Autodesk Fusion 360 part; units mm, degrees
(part 5 of 8)
  spline S134 degree 5 poles (58.96, -141.4145) (58.9068, -141.4906) (58.8007, -141.6428) (58.6419, -141.8712) (58.4312, -142.1762) (58.1694, -142.5582) (57.9092, -142.9408) (57.6506, -143.324) (57.3936, -143.708) (57.1382, -144.0925) (56.8845, -144.4778) (56.6323, -144.8637) (56.3819, -145.2503) (56.1331, -145.6375) (55.8859, -146.0254) (55.6405, -146.4139) (55.3968, -146.8031) (55.1548, -147.193) (54.9146, -147.5836) (54.6761, -147.9747) (54.4394, -148.3666) (54.2045, -148.7591) (53.9713, -149.1523) (53.74, -149.5462) (53.5106, -149.9407) (53.2829, -150.3358) (53.0572, -150.7317) (52.8333, -151.1282) (52.6114, -151.5253) (52.3914, -151.9232) (52.1734, -152.3217) (51.9573, -152.7208) (51.7432, -153.1207) (51.5311, -153.5212) (51.3211, -153.9223) (51.1132, -154.3242) (50.9074, -154.7267) (50.7037, -155.1299) (50.5021, -155.5337) (50.3027, -155.9383) (50.1056, -156.3435) (49.9107, -156.7494) (49.718, -157.156) (49.5277, -157.5633) (49.3397, -157.9713) (49.1542, -158.3799) (48.9711, -158.7893) (48.7905, -159.1994) (48.6124, -159.6102) (48.4369, -160.0216) (48.2641, -160.4338) (48.0939, -160.8467) (47.9263, -161.2604) (47.7616, -161.6747) (47.5997, -162.0898) (47.4409, -162.5056) (47.2851, -162.9223) (47.1327, -163.3396) (46.9836, -163.7578) (46.8379, -164.1768) (46.6955, -164.5965) (46.5565, -165.0171) (46.4209, -165.4384) (46.3021, -165.8187) (46.2122, -166.1152) (46.1493, -166.3273) (46.1121, -166.4549) (46.0997, -166.4977) knots -1 -1 -1 -1 -1 -1 -0.98571429 -0.97142857 -0.95714286 -0.94285714 -0.92857143 -0.91428571 -0.9 -0.88571429 -0.87142857 -0.85714286 -0.84285714 -0.82857143 -0.81428571 -0.8 -0.78571429 -0.77142857 -0.75714286 -0.74285714 -0.72857143 -0.71428571 -0.7 -0.68571429 -0.67142857 -0.65714286 -0.64285714 -0.62857143 -0.61428571 -0.6 -0.58571429 -0.57142857 -0.55714286 -0.54285714 -0.52857143 -0.51428571 -0.5 -0.48571429 -0.47142857 -0.45714286 -0.44285714 -0.42857143 -0.41428571 -0.4 -0.38571429 -0.37142857 -0.35714286 -0.34285714 -0.32857143 -0.31428571 -0.3 -0.28571429 -0.27142857 -0.25714286 -0.24285714 -0.22857143 -0.21428571 -0.2 -0.18571429 -0.17142857 -0.15714286 -0.14285714 -0.12857143 -0.11428571 -0.10707295 -0.10707295 -0.10707295 -0.10707295 -0.10707295 -0.10707295
  spline S135 degree 3 poles (44.3847, -167.6316) (44.5899, -167.6564) (44.798, -167.6408) (45.1965, -167.5309) (45.3832, -167.4375) (45.6787, -167.2088) (45.7938, -167.0864) (45.9817, -166.8102) (46.0532, -166.6581) (46.0997, -166.4977) knots 0 0 0 0 0.062015 0.062015 0.12403 0.12403 0.174133 0.174133 0.224236 0.224236 0.224236 0.224236
  arc A68 (44.3847, -167.6316) -> (36.0479, -166.7554) centre (11.949, -436.1388) ccw
  spline S136 degree 3 poles (34.6061, -165.2897) (34.6211, -165.4958) (34.6763, -165.6971) (34.8607, -166.0671) (34.9881, -166.2324) (35.2693, -166.4786) (35.4115, -166.5681) (35.7186, -166.6994) (35.8816, -166.7405) (36.0479, -166.7554) knots 0 0 0 0 0.062015 0.062015 0.12403 0.12403 0.174133 0.174133 0.224236 0.224236 0.224236 0.224236
  spline S137 degree 5 poles (34.6061, -165.2897) (34.6029, -165.2452) (34.593, -165.1127) (34.5756, -164.8921) (34.5493, -164.5834) (34.5122, -164.1867) (34.4672, -163.7464) (34.4186, -163.3062) (34.3666, -162.866) (34.3112, -162.4259) (34.2523, -161.9859) (34.19, -161.5459) (34.1243, -161.106) (34.0553, -160.6662) (33.9833, -160.2266) (33.9083, -159.787) (33.8304, -159.3476) (33.7498, -158.9083) (33.6664, -158.4692) (33.5803, -158.0302) (33.4916, -157.5914) (33.4002, -157.1527) (33.3062, -156.7143) (33.2096, -156.2759) (33.1106, -155.8378) (33.0091, -155.3998) (32.9052, -154.9621) (32.7989, -154.5245) (32.6903, -154.0872) (32.5794, -153.65) (32.4663, -153.2131) (32.3508, -152.7763) (32.2332, -152.3398) (32.1134, -151.9035) (31.9913, -151.4674) (31.8672, -151.0316) (31.7409, -150.596) (31.6125, -150.1606) (31.4821, -149.7255) (31.3496, -149.2906) (31.2151, -148.856) (31.0786, -148.4216) (30.9401, -147.9875) (30.7996, -147.5536) (30.6572, -147.12) (30.5128, -146.6867) (30.3665, -146.2537) (30.2183, -145.8209) (30.0683, -145.3884) (29.9163, -144.9561) (29.7625, -144.5242) (29.6069, -144.0925) (29.4494, -143.6611) (29.2902, -143.23) (29.1291, -142.7993) (28.9662, -142.3688) (28.8016, -141.9386) (28.6352, -141.5087) (28.4671, -141.0791) (28.2973, -140.6498) (28.1257, -140.2208) (27.9524, -139.7922) (27.7774, -139.3639) (27.6008, -138.9358) (27.4581, -138.5937) (27.3503, -138.3372) (27.2781, -138.1663) (27.242, -138.0808) knots 0.10707295 0.10707295 0.10707295 0.10707295 0.10707295 0.10707295 0.11428571 0.12857143 0.14285714 0.15714286 0.17142857 0.18571429 0.2 0.21428571 0.22857143 0.24285714 0.25714286 0.27142857 0.28571429 0.3 0.31428571 0.32857143 0.34285714 0.35714286 0.37142857 0.38571429 0.4 0.41428571 0.42857143 0.44285714 0.45714286 0.47142857 0.48571429 0.5 0.51428571 0.52857143 0.54285714 0.55714286 0.57142857 0.58571429 0.6 0.61428571 0.62857143 0.64285714 0.65714286 0.67142857 0.68571429 0.7 0.71428571 0.72857143 0.74285714 0.75714286 0.77142857 0.78571429 0.8 0.81428571 0.82857143 0.84285714 0.85714286 0.87142857 0.88571429 0.9 0.91428571 0.92857143 0.94285714 0.95714286 0.97142857 0.98571429 1 1 1 1 1 1
  arc A69 (27.242, -138.0808) -> (17.4848, -137.7401) centre (11.949, -436.1388) ccw
  spline S138 degree 5 poles (17.4848, -137.7401) (17.4427, -137.8228) (17.3588, -137.9883) (17.2334, -138.2366) (17.0672, -138.568) (16.8611, -138.9826) (16.6567, -139.3977) (16.4539, -139.8132) (16.2528, -140.2292) (16.0535, -140.6456) (15.8558, -141.0624) (15.6598, -141.4796) (15.4656, -141.8973) (15.2731, -142.3154) (15.0824, -142.7339) (14.8934, -143.1528) (14.7063, -143.5722) (14.5209, -143.9919) (14.3373, -144.4121) (14.1556, -144.8327) (13.9757, -145.2537) (13.7977, -145.6751) (13.6216, -146.0969) (13.4473, -146.5191) (13.275, -146.9417) (13.1046, -147.3647) (12.9361, -147.7881) (12.7697, -148.2119) (12.6052, -148.6361) (12.4427, -149.0606) (12.2822, -149.4856) (12.1238, -149.9109) (11.9674, -150.3367) (11.8132, -150.7628) (11.661, -151.1893) (11.511, -151.6162) (11.3632, -152.0434) (11.2176, -152.471) (11.0742, -152.899) (10.9331, -153.3274) (10.7943, -153.7561) (10.6578, -154.1852) (10.5236, -154.6146) (10.3918, -155.0444) (10.2624, -155.4746) (10.1355, -155.9051) (10.0112, -156.336) (9.8894, -156.7672) (9.7702, -157.1988) (9.6537, -157.6307) (9.5399, -158.0629) (9.4289, -158.4955) (9.3205, -158.9284) (9.2151, -159.3616) (9.1125, -159.7952) (9.0131, -160.2291) (8.9169, -160.6633) (8.824, -161.0979) (8.7345, -161.5327) (8.6485, -161.9679) (8.566, -162.4034) (8.4868, -162.8392) (8.4112, -163.2752) (8.3465, -163.6684) (8.2987, -163.9745) (8.266, -164.1933) (8.2469, -164.3248) (8.2406, -164.369) knots -1 -1 -1 -1 -1 -1 -0.98571429 -0.97142857 -0.95714286 -0.94285714 -0.92857143 -0.91428571 -0.9 -0.88571429 -0.87142857 -0.85714286 -0.84285714 -0.82857143 -0.81428571 -0.8 -0.78571429 -0.77142857 -0.75714286 -0.74285714 -0.72857143 -0.71428571 -0.7 -0.68571429 -0.67142857 -0.65714286 -0.64285714 -0.62857143 -0.61428571 -0.6 -0.58571429 -0.57142857 -0.55714286 -0.54285714 -0.52857143 -0.51428571 -0.5 -0.48571429 -0.47142857 -0.45714286 -0.44285714 -0.42857143 -0.41428571 -0.4 -0.38571429 -0.37142857 -0.35714286 -0.34285714 -0.32857143 -0.31428571 -0.3 -0.28571429 -0.27142857 -0.25714286 -0.24285714 -0.22857143 -0.21428571 -0.2 -0.18571429 -0.17142857 -0.15714286 -0.14285714 -0.12857143 -0.11428571 -0.10707295 -0.10707295 -0.10707295 -0.10707295 -0.10707295 -0.10707295
  spline S139 degree 3 poles (6.7, -165.7305) (6.9067, -165.7265) (7.1106, -165.6821) (7.49, -165.5178) (7.6618, -165.3994) (7.9226, -165.1317) (8.0196, -164.9945) (8.1672, -164.6948) (8.2168, -164.5343) (8.2406, -164.369) knots 0 0 0 0 0.062015 0.062015 0.12403 0.12403 0.174133 0.174133 0.224236 0.224236 0.224236 0.224236
  arc A70 (6.7, -165.7305) -> (-1.6775, -166.0231) centre (11.949, -436.1388) ccw
  spline S140 degree 3 poles (-3.3093, -164.7723) (-3.2657, -164.9744) (-3.1831, -165.166) (-2.949, -165.5068) (-2.7998, -165.6527) (-2.4871, -165.8573) (-2.3338, -165.9262) (-2.0114, -166.0135) (-1.8443, -166.0315) (-1.6775, -166.0231) knots 0 0 0 0 0.062015 0.062015 0.12403 0.12403 0.174133 0.174133 0.224236 0.224236 0.224236 0.224236
  spline S141 degree 5 poles (-3.3093, -164.7723) (-3.3187, -164.7287) (-3.3469, -164.5989) (-3.3948, -164.3828) (-3.4638, -164.0808) (-3.5558, -163.6931) (-3.6617, -163.2634) (-3.771, -162.8342) (-3.8838, -162.4055) (-3.9999, -161.9774) (-4.1195, -161.5499) (-4.2424, -161.1229) (-4.3687, -160.6964) (-4.4982, -160.2705) (-4.6307, -159.8451) (-4.7661, -159.4203) (-4.9044, -158.996) (-5.0454, -158.5722) (-5.1891, -158.149) (-5.3354, -157.7263) (-5.4844, -157.3041) (-5.6359, -156.8824) (-5.7901, -156.4612) (-5.9467, -156.0406) (-6.1057, -155.6205) (-6.2672, -155.201) (-6.431, -154.7819) (-6.5971, -154.3634) (-6.7655, -153.9454) (-6.9362, -153.528) (-7.109, -153.111) (-7.2841, -152.6946) (-7.4614, -152.2787) (-7.6408, -151.8633) (-7.8223, -151.4485) (-8.0059, -151.0342) (-8.1916, -150.6204) (-8.3793, -150.2071) (-8.569, -149.7944) (-8.7607, -149.3822) (-8.9544, -148.9705) (-9.15, -148.5593) (-9.3476, -148.1487) (-9.5471, -147.7386) (-9.7485, -147.3291) (-9.9518, -146.9201) (-10.1569, -146.5116) (-10.3639, -146.1036) (-10.5727, -145.6962) (-10.7833, -145.2893) (-10.9957, -144.883) (-11.2099, -144.4772) (-11.4259, -144.0719) (-11.6436, -143.6672) (-11.8631, -143.263) (-12.0843, -142.8594) (-12.3071, -142.4563) (-12.5317, -142.0537) (-12.758, -141.6517) (-12.986, -141.2502) (-13.2156, -140.8493) (-13.4468, -140.449) (-13.6797, -140.0492) (-13.9142, -139.6499) (-14.1031, -139.3309) (-14.2455, -139.0919) (-14.3408, -138.9327) (-14.3885, -138.8531) knots 0.10707295 0.10707295 0.10707295 0.10707295 0.10707295 0.10707295 0.11428571 0.12857143 0.14285714 0.15714286 0.17142857 0.18571429 0.2 0.21428571 0.22857143 0.24285714 0.25714286 0.27142857 0.28571429 0.3 0.31428571 0.32857143 0.34285714 0.35714286 0.37142857 0.38571429 0.4 0.41428571 0.42857143 0.44285714 0.45714286 0.47142857 0.48571429 0.5 0.51428571 0.52857143 0.54285714 0.55714286 0.57142857 0.58571429 0.6 0.61428571 0.62857143 0.64285714 0.65714286 0.67142857 0.68571429 0.7 0.71428571 0.72857143 0.74285714 0.75714286 0.77142857 0.78571429 0.8 0.81428571 0.82857143 0.84285714 0.85714286 0.87142857 0.88571429 0.9 0.91428571 0.92857143 0.94285714 0.95714286 0.97142857 0.98571429 1 1 1 1 1 1
  arc A71 (-14.3885, -138.8531) -> (-24.0982, -139.8737) centre (11.949, -436.1388) ccw
  spline S142 degree 5 poles (-24.0982, -139.8737) (-24.1283, -139.9614) (-24.1884, -140.137) (-24.278, -140.4003) (-24.3965, -140.7516) (-24.5428, -141.1909) (-24.6875, -141.6304) (-24.8305, -142.0701) (-24.9717, -142.51) (-25.1112, -142.9501) (-25.2489, -143.3903) (-25.3849, -143.8308) (-25.5191, -144.2714) (-25.6516, -144.7122) (-25.7822, -145.1532) (-25.911, -145.5944) (-26.038, -146.0357) (-26.1631, -146.4771) (-26.2864, -146.9188) (-26.4078, -147.3605) (-26.5274, -147.8025) (-26.645, -148.2445) (-26.7607, -148.6868) (-26.8745, -149.1291) (-26.9864, -149.5716) (-27.0962, -150.0142) (-27.2041, -150.4569) (-27.31, -150.8997) (-27.4139, -151.3427) (-27.5157, -151.7858) (-27.6155, -152.2289) (-27.7131, -152.6722) (-27.8087, -153.1155) (-27.9022, -153.559) (-27.9935, -154.0025) (-28.0826, -154.4461) (-28.1695, -154.8897) (-28.2542, -155.3335) (-28.3366, -155.7772) (-28.4167, -156.2211) (-28.4945, -156.6649) (-28.57, -157.1088) (-28.6431, -157.5528) (-28.7138, -157.9968) (-28.7821, -158.4407) (-28.8478, -158.8847) (-28.911, -159.3287) (-28.9716, -159.7727) (-29.0295, -160.2166) (-29.0847, -160.6605) (-29.1373, -161.1044) (-29.1871, -161.5482) (-29.2341, -161.992) (-29.2783, -162.4357) (-29.3195, -162.8793) (-29.3576, -163.3228) (-29.3924, -163.7662) (-29.4239, -164.2095) (-29.452, -164.6525) (-29.4766, -165.0954) (-29.4977, -165.5382) (-29.5154, -165.9807) (-29.5296, -166.4231) (-29.539, -166.8215) (-29.5437, -167.1312) (-29.5456, -167.3525) (-29.5462, -167.4853) (-29.5464, -167.5299) knots -1 -1 -1 -1 -1 -1 -0.98571429 -0.97142857 -0.95714286 -0.94285714 -0.92857143 -0.91428571 -0.9 -0.88571429 -0.87142857 -0.85714286 -0.84285714 -0.82857143 -0.81428571 -0.8 -0.78571429 -0.77142857 -0.75714286 -0.74285714 -0.72857143 -0.71428571 -0.7 -0.68571429 -0.67142857 -0.65714286 -0.64285714 -0.62857143 -0.61428571 -0.6 -0.58571429 -0.57142857 -0.55714286 -0.54285714 -0.52857143 -0.51428571 -0.5 -0.48571429 -0.47142857 -0.45714286 -0.44285714 -0.42857143 -0.41428571 -0.4 -0.38571429 -0.37142857 -0.35714286 -0.34285714 -0.32857143 -0.31428571 -0.3 -0.28571429 -0.27142857 -0.25714286 -0.24285714 -0.22857143 -0.21428571 -0.2 -0.18571429 -0.17142857 -0.15714286 -0.14285714 -0.12857143 -0.11428571 -0.10707295 -0.10707295 -0.10707295 -0.10707295 -0.10707295 -0.10707295
  spline S143 degree 3 poles (-30.8825, -169.0926) (-30.6783, -169.0599) (-30.4826, -168.9876) (-30.1298, -168.772) (-29.9761, -168.6308) (-29.7551, -168.3295) (-29.6782, -168.1801) (-29.5737, -167.8628) (-29.5469, -167.6969) (-29.5464, -167.5299) knots 0 0 0 0 0.062015 0.062015 0.12403 0.12403 0.174133 0.174133 0.224236 0.224236 0.224236 0.224236
  arc A72 (-30.8825, -169.0926) -> (-39.1377, -170.5482) centre (11.949, -436.1388) ccw
  spline S144 degree 3 poles (-40.9277, -169.5368) (-40.8564, -169.7308) (-40.7479, -169.9091) (-40.4687, -170.2139) (-40.3007, -170.3377) (-39.9625, -170.4968) (-39.8011, -170.5436) (-39.4697, -170.5853) (-39.3017, -170.5798) (-39.1377, -170.5482) knots 0 0 0 0 0.062015 0.062015 0.12403 0.12403 0.174133 0.174133 0.224236 0.224236 0.224236 0.224236
  spline S145 degree 5 poles (-40.9277, -169.5368) (-40.9431, -169.4949) (-40.9891, -169.3703) (-41.0666, -169.163) (-41.177, -168.8735) (-41.322, -168.5024) (-41.4866, -168.0916) (-41.6547, -167.6818) (-41.826, -167.273) (-42.0006, -166.8652) (-42.1785, -166.4585) (-42.3597, -166.0527) (-42.5441, -165.648) (-42.7315, -165.2442) (-42.922, -164.8415) (-43.1152, -164.4396) (-43.3112, -164.0387) (-43.5098, -163.6386) (-43.711, -163.2395) (-43.9147, -162.8413) (-44.121, -162.4439) (-44.3298, -162.0474) (-44.541, -161.6519) (-44.7546, -161.2571) (-44.9706, -160.8633) (-45.1889, -160.4703) (-45.4094, -160.0781) (-45.6322, -159.6868) (-45.8571, -159.2963) (-46.0842, -158.9066) (-46.3134, -158.5178) (-46.5448, -158.1298) (-46.7782, -157.7426) (-47.0136, -157.3562) (-47.2511, -156.9707) (-47.4906, -156.586) (-47.732, -156.202) (-47.9754, -155.8189) (-48.2208, -155.4366) (-48.468, -155.0551) (-48.7171, -154.6744) (-48.968, -154.2945) (-49.2208, -153.9153) (-49.4755, -153.537) (-49.7319, -153.1595) (-49.9901, -152.7827) (-50.2501, -152.4068) (-50.5119, -152.0316) (-50.7753, -151.6572) (-51.0405, -151.2836) (-51.3074, -150.9108) (-51.576, -150.5387) (-51.8463, -150.1674) (-52.1182, -149.797) (-52.3918, -149.4273) (-52.667, -149.0583) (-52.9438, -148.6902) (-53.2222, -148.3228) (-53.5022, -147.9562) (-53.7838, -147.5904) (-54.067, -147.2253) (-54.3517, -146.861) (-54.638, -146.4975) (-54.9258, -146.1348) (-55.1572, -145.8452) (-55.3315, -145.6283) (-55.448, -145.4839) (-55.5064, -145.4118) knots 0.10707295 0.10707295 0.10707295 0.10707295 0.10707295 0.10707295 0.11428571 0.12857143 0.14285714 0.15714286 0.17142857 0.18571429 0.2 0.21428571 0.22857143 0.24285714 0.25714286 0.27142857 0.28571429 0.3 0.31428571 0.32857143 0.34285714 0.35714286 0.37142857 0.38571429 0.4 0.41428571 0.42857143 0.44285714 0.45714286 0.47142857 0.48571429 0.5 0.51428571 0.52857143 0.54285714 0.55714286 0.57142857 0.58571429 0.6 0.61428571 0.62857143 0.64285714 0.65714286 0.67142857 0.68571429 0.7 0.71428571 0.72857143 0.74285714 0.75714286 0.77142857 0.78571429 0.8 0.81428571 0.82857143 0.84285714 0.85714286 0.87142857 0.88571429 0.9 0.91428571 0.92857143 0.94285714 0.95714286 0.97142857 0.98571429 1 1 1 1 1 1
  arc A73 (-55.5064, -145.4118) -> (-64.9795, -147.7737) centre (11.949, -436.1388) ccw
  spline S146 degree 5 poles (-64.9795, -147.7737) (-64.9971, -147.8648) (-65.0322, -148.047) (-65.0843, -148.3203) (-65.1527, -148.6846) (-65.2365, -149.14) (-65.3186, -149.5954) (-65.399, -150.0507) (-65.4776, -150.5059) (-65.5545, -150.9611) (-65.6296, -151.4163) (-65.703, -151.8714) (-65.7746, -152.3264) (-65.8444, -152.7814) (-65.9123, -153.2362) (-65.9785, -153.691) (-66.0428, -154.1457) (-66.1053, -154.6003) (-66.1659, -155.0548) (-66.2247, -155.5092) (-66.2816, -155.9634) (-66.3365, -156.4176) (-66.3896, -156.8716) (-66.4407, -157.3254) (-66.4899, -157.7792) (-66.5371, -158.2328) (-66.5823, -158.6862) (-66.6255, -159.1395) (-66.6668, -159.5926) (-66.7059, -160.0455) (-66.743, -160.4982) (-66.7781, -160.9508) (-66.811, -161.4031) (-66.8418, -161.8552) (-66.8705, -162.3071) (-66.897, -162.7588) (-66.9214, -163.2102) (-66.9435, -163.6614) (-66.9633, -164.1124) (-66.9809, -164.563) (-66.9962, -165.0134) (-67.0092, -165.4635) (-67.0198, -165.9133) (-67.028, -166.3628) (-67.0338, -166.8119) (-67.0371, -167.2608) (-67.0379, -167.7092) (-67.0361, -168.1573) (-67.0316, -168.605) (-67.0246, -169.0522) (-67.0148, -169.4991) (-67.0024, -169.9456) (-66.9872, -170.3916) (-66.9692, -170.8371) (-66.9482, -171.2821) (-66.9242, -171.7266) (-66.897, -172.1706) (-66.8665, -172.6139) (-66.8326, -173.0565) (-66.7953, -173.4985) (-66.7547, -173.9399) (-66.7106, -174.3806) (-66.6631, -174.8207) (-66.617, -175.2164) (-66.5785, -175.5238) (-66.5496, -175.7432) (-66.5317, -175.8749) (-66.5257, -175.919) knots -1 -1 -1 -1 -1 -1 -0.98571429 -0.97142857 -0.95714286 -0.94285714 -0.92857143 -0.91428571 -0.9 -0.88571429 -0.87142857 -0.85714286 -0.84285714 -0.82857143 -0.81428571 -0.8 -0.78571429 -0.77142857 -0.75714286 -0.74285714 -0.72857143 -0.71428571 -0.7 -0.68571429 -0.67142857 -0.65714286 -0.64285714 -0.62857143 -0.61428571 -0.6 -0.58571429 -0.57142857 -0.55714286 -0.54285714 -0.52857143 -0.51428571 -0.5 -0.48571429 -0.47142857 -0.45714286 -0.44285714 -0.42857143 -0.41428571 -0.4 -0.38571429 -0.37142857 -0.35714286 -0.34285714 -0.32857143 -0.31428571 -0.3 -0.28571429 -0.27142857 -0.25714286 -0.24285714 -0.22857143 -0.21428571 -0.2 -0.18571429 -0.17142857 -0.15714286 -0.14285714 -0.12857143 -0.11428571 -0.10707295 -0.10707295 -0.10707295 -0.10707295 -0.10707295 -0.10707295
  spline S147 degree 3 poles (-67.6313, -177.6525) (-67.4337, -177.5917) (-67.2499, -177.4928) (-66.9305, -177.2303) (-66.798, -177.0691) (-66.6211, -176.7399) (-66.5657, -176.5812) (-66.5064, -176.2525) (-66.5029, -176.0845) (-66.5257, -175.919) knots 0 0 0 0 0.062015 0.062015 0.12403 0.12403 0.174133 0.174133 0.224236 0.224236 0.224236 0.224236
  arc A74 (-67.6313, -177.6525) -> (-75.6036, -180.2429) centre (11.949, -436.1388) ccw
  spline S148 degree 3 poles (-77.517, -179.4903) (-77.4194, -179.6726) (-77.2871, -179.834) (-76.9682, -180.097) (-76.7845, -180.1962) (-76.4275, -180.3067) (-76.2612, -180.3306) (-75.9272, -180.3257) (-75.7616, -180.2969) (-75.6036, -180.2429) knots 0 0 0 0 0.062015 0.062015 0.12403 0.12403 0.174133 0.174133 0.224236 0.224236 0.224236 0.224236
  spline S149 degree 5 poles (-77.517, -179.4903) (-77.538, -179.451) (-77.6009, -179.334) (-77.7065, -179.1395) (-77.8561, -178.8683) (-78.0514, -178.5209) (-78.2716, -178.137) (-78.495, -177.7546) (-78.7215, -177.3736) (-78.9512, -176.9941) (-79.184, -176.6161) (-79.4198, -176.2395) (-79.6588, -175.8644) (-79.9006, -175.4906) (-80.1453, -175.1183) (-80.3926, -174.7472) (-80.6424, -174.3775) (-80.8948, -174.009) (-81.1495, -173.6417) (-81.4067, -173.2757) (-81.6663, -172.9109) (-81.9282, -172.5474) (-82.1924, -172.185) (-82.4589, -171.8239) (-82.7276, -171.4639) (-82.9985, -171.1051) (-83.2714, -170.7474) (-83.5465, -170.3909) (-83.8236, -170.0355) (-84.1027, -169.6813) (-84.3838, -169.3281) (-84.6669, -168.9761) (-84.9519, -168.6252) (-85.2388, -168.2754) (-85.5277, -167.9266) (-85.8184, -167.579) (-86.1109, -167.2324) (-86.4052, -166.8869) (-86.7014, -166.5424) (-86.9993, -166.199) (-87.2989, -165.8567) (-87.6003, -165.5154) (-87.9034, -165.1751) (-88.2083, -164.8359) (-88.5147, -164.4977) (-88.8229, -164.1606) (-89.1327, -163.8245) (-89.4441, -163.4894) (-89.7571, -163.1553) (-90.0717, -162.8222) (-90.3879, -162.4902) (-90.7056, -162.1591) (-91.0249, -161.8291) (-91.3458, -161.5001) (-91.6681, -161.172) (-91.992, -160.845) (-92.3174, -160.5189) (-92.6442, -160.1939) (-92.9725, -159.8698) (-93.3023, -159.5467) (-93.6335, -159.2246) (-93.9662, -158.9035) (-94.3002, -158.5834) (-94.6357, -158.2642) (-94.9052, -158.0097) (-95.108, -157.8192) (-95.2435, -157.6924) (-95.3113, -157.6291) knots 0.10707295 0.10707295 0.10707295 0.10707295 0.10707295 0.10707295 0.11428571 0.12857143 0.14285714 0.15714286 0.17142857 0.18571429 0.2 0.21428571 0.22857143 0.24285714 0.25714286 0.27142857 0.28571429 0.3 0.31428571 0.32857143 0.34285714 0.35714286 0.37142857 0.38571429 0.4 0.41428571 0.42857143 0.44285714 0.45714286 0.47142857 0.48571429 0.5 0.51428571 0.52857143 0.54285714 0.55714286 0.57142857 0.58571429 0.6 0.61428571 0.62857143 0.64285714 0.65714286 0.67142857 0.68571429 0.7 0.71428571 0.72857143 0.74285714 0.75714286 0.77142857 0.78571429 0.8 0.81428571 0.82857143 0.84285714 0.85714286 0.87142857 0.88571429 0.9 0.91428571 0.92857143 0.94285714 0.95714286 0.97142857 0.98571429 1 1 1 1 1 1
  arc A75 (-95.3113, -157.6291) -> (-104.3635, -161.2864) centre (11.949, -436.1388) ccw
  spline S150 degree 5 poles (-104.3635, -161.2864) (-104.3683, -161.3791) (-104.3776, -161.5644) (-104.3912, -161.8423) (-104.4082, -162.2126) (-104.4278, -162.6752) (-104.4458, -163.1376) (-104.462, -163.5996) (-104.4765, -164.0614) (-104.4893, -164.5229) (-104.5003, -164.9841) (-104.5097, -165.4449) (-104.5172, -165.9055) (-104.523, -166.3657) (-104.527, -166.8256) (-104.5293, -167.2852) (-104.5297, -167.7444) (-104.5283, -168.2033) (-104.5251, -168.6618) (-104.52, -169.1199) (-104.5131, -169.5777) (-104.5043, -170.035) (-104.4937, -170.492) (-104.4811, -170.9486) (-104.4667, -171.4047) (-104.4503, -171.8605) (-104.432, -172.3158) (-104.4117, -172.7707) (-104.3895, -173.2251) (-104.3652, -173.6791) (-104.339, -174.1325) (-104.3107, -174.5856) (-104.2803, -175.0381) (-104.248, -175.4901) (-104.2135, -175.9416) (-104.1769, -176.3926) (-104.1381, -176.843) (-104.0972, -177.2929) (-104.0541, -177.7422) (-104.0088, -178.1909) (-103.9613, -178.639) (-103.9115, -179.0865) (-103.8594, -179.5334) (-103.8049, -179.9797) (-103.7482, -180.4253) (-103.689, -180.8702) (-103.6273, -181.3144) (-103.5632, -181.7579) (-103.4965, -182.2006) (-103.4273, -182.6425) (-103.3554, -183.0837) (-103.281, -183.524) (-103.2038, -183.9636) (-103.124, -184.4023) (-103.0413, -184.8401) (-102.9557, -185.2769) (-102.8669, -185.7127) (-102.7751, -186.1475) (-102.6799, -186.5811) (-102.5815, -187.0136) (-102.4798, -187.4451) (-102.3748, -187.8753) (-102.2665, -188.3045) (-102.1657, -188.69) (-102.0849, -188.989) (-102.0258, -189.2023) (-101.9897, -189.3302) (-101.9775, -189.373) knots -1 -1 -1 -1 -1 -1 -0.98571429 -0.97142857 -0.95714286 -0.94285714 -0.92857143 -0.91428571 -0.9 -0.88571429 -0.87142857 -0.85714286 -0.84285714 -0.82857143 -0.81428571 -0.8 -0.78571429 -0.77142857 -0.75714286 -0.74285714 -0.72857143 -0.71428571 -0.7 -0.68571429 -0.67142857 -0.65714286 -0.64285714 -0.62857143 -0.61428571 -0.6 -0.58571429 -0.57142857 -0.55714286 -0.54285714 -0.52857143 -0.51428571 -0.5 -0.48571429 -0.47142857 -0.45714286 -0.44285714 -0.42857143 -0.41428571 -0.4 -0.38571429 -0.37142857 -0.35714286 -0.34285714 -0.32857143 -0.31428571 -0.3 -0.28571429 -0.27142857 -0.25714286 -0.24285714 -0.22857143 -0.21428571 -0.2 -0.18571429 -0.17142857 -0.15714286 -0.14285714 -0.12857143 -0.11428571 -0.10707295 -0.10707295 -0.10707295 -0.10707295 -0.10707295 -0.10707295
  spline S151 degree 3 poles (-102.8311, -191.2435) (-102.644, -191.1558) (-102.4757, -191.0323) (-102.196, -190.7279) (-102.0872, -190.5498) (-101.9578, -190.1992) (-101.925, -190.0344) (-101.9121, -189.7006) (-101.932, -189.5337) (-101.9775, -189.373) knots 0 0 0 0 0.062015 0.062015 0.12403 0.12403 0.174133 0.174133 0.224236 0.224236 0.224236 0.224236
  arc A76 (-102.8311, -191.2435) -> (-110.3654, -194.9182) centre (11.949, -436.1388) ccw
  spline S152 degree 3 poles (-112.3648, -194.4393) (-112.2428, -194.6061) (-112.0894, -194.7476) (-111.737, -194.9637) (-111.5413, -195.0363) (-111.1724, -195.0961) (-111.0043, -195.0966) (-110.6743, -195.0453) (-110.5144, -194.9937) (-110.3654, -194.9182) knots 0 0 0 0 0.062015 0.062015 0.12403 0.12403 0.174133 0.174133 0.224236 0.224236 0.224236 0.224236
  spline S153 degree 5 poles (-112.3648, -194.4393) (-112.3912, -194.4033) (-112.4697, -194.2961) (-112.6013, -194.1183) (-112.7872, -193.8704) (-113.029, -193.5537) (-113.3005, -193.2041) (-113.5749, -192.8565) (-113.8523, -192.5108) (-114.1325, -192.1669) (-114.4156, -191.825) (-114.7016, -191.4849) (-114.9905, -191.1467) (-115.282, -190.8102) (-115.576, -190.4756) (-115.8726, -190.1425) (-116.1715, -189.8111) (-116.4726, -189.4814) (-116.776, -189.1531) (-117.0817, -188.8265) (-117.3895, -188.5014) (-117.6994, -188.1778) (-118.0115, -187.8558) (-118.3257, -187.5352) (-118.6418, -187.2161) (-118.96, -186.8985) (-119.2801, -186.5823) (-119.6021, -186.2676) (-119.9259, -185.9542) (-120.2516, -185.6422) (-120.5791, -185.3317) (-120.9085, -185.0225) (-121.2396, -184.7146) (-121.5724, -184.4081) (-121.907, -184.103) (-122.2432, -183.7991) (-122.5811, -183.4966) (-122.9207, -183.1955) (-123.2619, -182.8956) (-123.6047, -182.597) (-123.9491, -182.2997) (-124.295, -182.0036) (-124.6425, -181.7089) (-124.9916, -181.4154) (-125.3422, -181.1232) (-125.6942, -180.8322) (-126.0478, -180.5425) (-126.4028, -180.254) (-126.7592, -179.9667) (-127.1171, -179.6807) (-127.4765, -179.3958) (-127.8372, -179.1122) (-128.1993, -178.8299) (-128.5628, -178.5487) (-128.9277, -178.2687) (-129.2939, -177.9899) (-129.6615, -177.7123) (-130.0304, -177.4359) (-130.4007, -177.1607) (-130.7722, -176.8867) (-131.145, -176.6138) (-131.5191, -176.3421) (-131.8945, -176.0716) (-132.2711, -175.8022) (-132.5734, -175.5877) (-132.8007, -175.4273) (-132.9525, -175.3206) (-133.0285, -175.2673) knots 0.10707295 0.10707295 0.10707295 0.10707295 0.10707295 0.10707295 0.11428571 0.12857143 0.14285714 0.15714286 0.17142857 0.18571429 0.2 0.21428571 0.22857143 0.24285714 0.25714286 0.27142857 0.28571429 0.3 0.31428571 0.32857143 0.34285714 0.35714286 0.37142857 0.38571429 0.4 0.41428571 0.42857143 0.44285714 0.45714286 0.47142857 0.48571429 0.5 0.51428571 0.52857143 0.54285714 0.55714286 0.57142857 0.58571429 0.6 0.61428571 0.62857143 0.64285714 0.65714286 0.67142857 0.68571429 0.7 0.71428571 0.72857143 0.74285714 0.75714286 0.77142857 0.78571429 0.8 0.81428571 0.82857143 0.84285714 0.85714286 0.87142857 0.88571429 0.9 0.91428571 0.92857143 0.94285714 0.95714286 0.97142857 0.98571429 1 1 1 1 1 1
  arc A77 (-133.0285, -175.2673) -> (-141.4836, -180.1488) centre (11.949, -436.1388) ccw
  spline S154 degree 5 poles (-141.4836, -180.1488) (-141.4754, -180.2413) (-141.4589, -180.4261) (-141.4337, -180.7031) (-141.399, -181.0722) (-141.354, -181.5331) (-141.3075, -181.9934) (-141.2592, -182.4532) (-141.2093, -182.9125) (-141.1577, -183.3713) (-141.1045, -183.8295) (-141.0496, -184.2872) (-140.993, -184.7444) (-140.9347, -185.2009) (-140.8746, -185.6569) (-140.8129, -186.1123) (-140.7494, -186.5671) (-140.6841, -187.0213) (-140.6172, -187.4749) (-140.5484, -187.9279) (-140.4778, -188.3802) (-140.4055, -188.8319) (-140.3314, -189.283) (-140.2554, -189.7333) (-140.1776, -190.1831) (-140.0979, -190.6321) (-140.0164, -191.0804) (-139.9331, -191.528) (-139.8478, -191.9749) (-139.7606, -192.4211) (-139.6715, -192.8665) (-139.5804, -193.3112) (-139.4874, -193.7551) (-139.3924, -194.1982) (-139.2954, -194.6405) (-139.1964, -195.082) (-139.0954, -195.5227) (-138.9922, -195.9625) (-138.887, -196.4014) (-138.7797, -196.8394) (-138.6703, -197.2766) (-138.5587, -197.7128) (-138.4449, -198.1481) (-138.3289, -198.5825) (-138.2106, -199.0158) (-138.0901, -199.4481) (-137.9672, -199.8794) (-137.842, -200.3097) (-137.7144, -200.7388) (-137.5843, -201.1668) (-137.4518, -201.5937) (-137.3167, -202.0194) (-137.1792, -202.4439) (-137.039, -202.8672) (-136.8962, -203.2892) (-136.7506, -203.7099) (-136.6021, -204.1291) (-136.4506, -204.5469) (-136.296, -204.9631) (-136.1384, -205.3777) (-135.9776, -205.7907) (-135.8138, -206.2022) (-135.6468, -206.6121) (-135.4934, -206.9799) (-135.3717, -207.2647) (-135.2835, -207.4677) (-135.23, -207.5893) (-135.212, -207.6301) knots -1 -1 -1 -1 -1 -1 -0.98571429 -0.97142857 -0.95714286 -0.94285714 -0.92857143 -0.91428571 -0.9 -0.88571429 -0.87142857 -0.85714286 -0.84285714 -0.82857143 -0.81428571 -0.8 -0.78571429 -0.77142857 -0.75714286 -0.74285714 -0.72857143 -0.71428571 -0.7 -0.68571429 -0.67142857 -0.65714286 -0.64285714 -0.62857143 -0.61428571 -0.6 -0.58571429 -0.57142857 -0.55714286 -0.54285714 -0.52857143 -0.51428571 -0.5 -0.48571429 -0.47142857 -0.45714286 -0.44285714 -0.42857143 -0.41428571 -0.4 -0.38571429 -0.37142857 -0.35714286 -0.34285714 -0.32857143 -0.31428571 -0.3 -0.28571429 -0.27142857 -0.25714286 -0.24285714 -0.22857143 -0.21428571 -0.2 -0.18571429 -0.17142857 -0.15714286 -0.14285714 -0.12857143 -0.11428571 -0.10707295 -0.10707295 -0.10707295 -0.10707295 -0.10707295 -0.10707295
  spline S155 degree 3 poles (-135.7969, -209.6011) (-135.6238, -209.4882) (-135.4744, -209.3425) (-135.2397, -209.0021) (-135.1568, -208.8106) (-135.0774, -208.4454) (-135.0679, -208.2776) (-135.1016, -207.9453) (-135.1445, -207.7828) (-135.212, -207.6301) knots 0 0 0 0 0.062015 0.062015 0.12403 0.12403 0.174133 0.174133 0.224236 0.224236 0.224236 0.224236
  arc A78 (-135.7969, -209.6011) -> (-142.7465, -214.2886) centre (11.949, -436.1388) ccw
  spline S156 degree 3 poles (-144.7931, -214.0926) (-144.6491, -214.2409) (-144.4774, -214.3596) (-144.0983, -214.5246) (-143.8945, -214.5692) (-143.5208, -214.5771) (-143.3544, -214.5542) (-143.0347, -214.4574) (-142.8835, -214.3841) (-142.7465, -214.2886) knots 0 0 0 0 0.062015 0.062015 0.12403 0.12403 0.174133 0.174133 0.224236 0.224236 0.224236 0.224236
  spline S157 degree 5 poles (-144.7931, -214.0926) (-144.8242, -214.0606) (-144.9169, -213.9655) (-145.072, -213.8076) (-145.2905, -213.5881) (-145.574, -213.3081) (-145.8915, -212.9997) (-146.2117, -212.6937) (-146.5344, -212.3899) (-146.8598, -212.0884) (-147.1878, -211.7892) (-147.5183, -211.4922) (-147.8514, -211.1975) (-148.1869, -210.9049) (-148.5247, -210.6144) (-148.8647, -210.3259) (-149.2068, -210.0393) (-149.5509, -209.7546) (-149.897, -209.4719) (-150.2452, -209.1909) (-150.5952, -208.9118) (-150.9472, -208.6345) (-151.3011, -208.3591) (-151.6568, -208.0853) (-152.0143, -207.8134) (-152.3735, -207.5431) (-152.7345, -207.2746) (-153.0972, -207.0077) (-153.4615, -206.7424) (-153.8274, -206.4788) (-154.195, -206.2168) (-154.5641, -205.9565) (-154.9349, -205.6977) (-155.3071, -205.4405) (-155.6809, -205.1849) (-156.0561, -204.9308) (-156.4329, -204.6783) (-156.811, -204.4273) (-157.1907, -204.1778) (-157.5717, -203.9299) (-157.9541, -203.6834) (-158.3379, -203.4384) (-158.723, -203.1949) (-159.1095, -202.9528) (-159.4974, -202.7122) (-159.8865, -202.4731) (-160.2769, -202.2353) (-160.6686, -201.9991) (-161.0616, -201.7642) (-161.4558, -201.5308) (-161.8513, -201.2987) (-162.248, -201.0681) (-162.6459, -200.8388) (-163.045, -200.611) (-163.4453, -200.3845) (-163.8468, -200.1594) (-164.2494, -199.9357) (-164.6532, -199.7133) (-165.0581, -199.4923) (-165.4641, -199.2726) (-165.8713, -199.0543) (-166.2796, -198.8373) (-166.6889, -198.6217) (-167.0994, -198.4074) (-167.4286, -198.237) (-167.6761, -198.1098) (-167.8412, -198.0252) (-167.9238, -197.983) knots 0.10707295 0.10707295 0.10707295 0.10707295 0.10707295 0.10707295 0.11428571 0.12857143 0.14285714 0.15714286 0.17142857 0.18571429 0.2 0.21428571 0.22857143 0.24285714 0.25714286 0.27142857 0.28571429 0.3 0.31428571 0.32857143 0.34285714 0.35714286 0.37142857 0.38571429 0.4 0.41428571 0.42857143 0.44285714 0.45714286 0.47142857 0.48571429 0.5 0.51428571 0.52857143 0.54285714 0.55714286 0.57142857 0.58571429 0.6 0.61428571 0.62857143 0.64285714 0.65714286 0.67142857 0.68571429 0.7 0.71428571 0.72857143 0.74285714 0.75714286 0.77142857 0.78571429 0.8 0.81428571 0.82857143 0.84285714 0.85714286 0.87142857 0.88571429 0.9 0.91428571 0.92857143 0.94285714 0.95714286 0.97142857 0.98571429 1 1 1 1 1 1
  arc A79 (-167.9238, -197.983) -> (-175.6173, -203.9938) centre (11.949, -436.1388) ccw
  spline S158 degree 5 poles (-175.6173, -203.9938) (-175.5964, -204.0842) (-175.5543, -204.2649) (-175.4907, -204.5357) (-175.405, -204.8964) (-175.2964, -205.3465) (-175.1862, -205.7959) (-175.0744, -206.2445) (-174.9611, -206.6924) (-174.8462, -207.1396) (-174.7297, -207.5859) (-174.6116, -208.0315) (-174.4919, -208.4763) (-174.3706, -208.9203) (-174.2477, -209.3635) (-174.1232, -209.8059) (-173.997, -210.2474) (-173.8692, -210.6881) (-173.7397, -211.128) (-173.6086, -211.567) (-173.4758, -212.0051) (-173.3413, -212.4423) (-173.2051, -212.8787) (-173.0672, -213.3141) (-172.9275, -213.7486) (-172.7862, -214.1822) (-172.6431, -214.6148) (-172.4982, -215.0465) (-172.3515, -215.4772) (-172.2031, -215.9068) (-172.0529, -216.3355) (-171.9008, -216.7632) (-171.7469, -217.1898) (-171.5912, -217.6154) (-171.4336, -218.0399) (-171.2741, -218.4633) (-171.1127, -218.8856) (-170.9494, -219.3068) (-170.7841, -219.7268) (-170.6169, -220.1457) (-170.4476, -220.5633) (-170.2764, -220.9798) (-170.1031, -221.395) (-169.9278, -221.809) (-169.7504, -222.2217) (-169.5709, -222.633) (-169.3892, -223.043) (-169.2053, -223.4516) (-169.0192, -223.8588) (-168.8308, -224.2645) (-168.6402, -224.6688) (-168.4472, -225.0716) (-168.2519, -225.4728) (-168.0542, -225.8725) (-167.8541, -226.2706) (-167.6513, -226.6669) (-167.4459, -227.0614) (-167.2378, -227.4539) (-167.0268, -227.8446) (-166.8129, -228.2332) (-166.5963, -228.6199) (-166.3768, -229.0046) (-166.1544, -229.3872) (-165.9512, -229.73) (-165.7911, -229.9952) (-165.6755, -230.1839) (-165.6056, -230.2969) (-165.5821, -230.3347) knots -1 -1 -1 -1 -1 -1 -0.98571429 -0.97142857 -0.95714286 -0.94285714 -0.92857143 -0.91428571 -0.9 -0.88571429 -0.87142857 -0.85714286 -0.84285714 -0.82857143 -0.81428571 -0.8 -0.78571429 -0.77142857 -0.75714286 -0.74285714 -0.72857143 -0.71428571 -0.7 -0.68571429 -0.67142857 -0.65714286 -0.64285714 -0.62857143 -0.61428571 -0.6 -0.58571429 -0.57142857 -0.55714286 -0.54285714 -0.52857143 -0.51428571 -0.5 -0.48571429 -0.47142857 -0.45714286 -0.44285714 -0.42857143 -0.41428571 -0.4 -0.38571429 -0.37142857 -0.35714286 -0.34285714 -0.32857143 -0.31428571 -0.3 -0.28571429 -0.27142857 -0.25714286 -0.24285714 -0.22857143 -0.21428571 -0.2 -0.18571429 -0.17142857 -0.15714286 -0.14285714 -0.12857143 -0.11428571 -0.10707295 -0.10707295 -0.10707295 -0.10707295 -0.10707295 -0.10707295
  spline S159 degree 3 poles (-165.887, -232.368) (-165.7313, -232.2321) (-165.6036, -232.067) (-165.4186, -231.6973) (-165.3631, -231.4961) (-165.3353, -231.1234) (-165.3493, -230.956) (-165.4289, -230.6316) (-165.494, -230.4766) (-165.5821, -230.3347) knots 0 0 0 0 0.062015 0.062015 0.12403 0.12403 0.174133 0.174133 0.224236 0.224236 0.224236 0.224236
  arc A80 (-165.887, -232.368) -> (-172.1165, -237.9771) centre (11.949, -436.1388) ccw
  spline S160 degree 3 poles (-174.1705, -238.0678) (-174.0073, -238.1946) (-173.8208, -238.2883) (-173.4224, -238.3989) (-173.2143, -238.4148) (-172.8432, -238.3705) (-172.6816, -238.3247) (-172.3785, -238.1844) (-172.2389, -238.0907) (-172.1165, -237.9771) knots 0 0 0 0 0.062015 0.062015 0.12403 0.12403 0.174133 0.174133 0.224236 0.224236 0.224236 0.224236
  spline S161 degree 5 poles (-174.1705, -238.0678) (-174.2058, -238.0405) (-174.3108, -237.9592) (-174.4864, -237.8245) (-174.7334, -237.6375) (-175.053, -237.3996) (-175.4104, -237.1384) (-175.77, -236.8799) (-176.1319, -236.624) (-176.4961, -236.3708) (-176.8625, -236.1201) (-177.2312, -235.872) (-177.602, -235.6265) (-177.975, -235.3835) (-178.3499, -235.1428) (-178.7267, -234.9044) (-179.1054, -234.6682) (-179.4858, -234.4342) (-179.8679, -234.2024) (-180.2517, -233.9726) (-180.6372, -233.745) (-181.0244, -233.5194) (-181.4131, -233.2958) (-181.8035, -233.0743) (-182.1954, -232.8547) (-182.5887, -232.6371) (-182.9836, -232.4214) (-183.3798, -232.2075) (-183.7775, -231.9956) (-184.1766, -231.7855) (-184.577, -231.5772) (-184.9788, -231.3708) (-185.382, -231.1661) (-185.7864, -230.9632) (-186.1921, -230.7621) (-186.599, -230.5627) (-187.0073, -230.3651) (-187.4167, -230.1692) (-187.8273, -229.975) (-188.2391, -229.7824) (-188.6521, -229.5916) (-189.0663, -229.4024) (-189.4816, -229.2148) (-189.898, -229.0289) (-190.3155, -228.8446) (-190.7342, -228.662) (-191.1539, -228.4809) (-191.5747, -228.3014) (-191.9965, -228.1235) (-192.4194, -227.9472) (-192.8433, -227.7725) (-193.2682, -227.5993) (-193.6942, -227.4277) (-194.1211, -227.2576) (-194.549, -227.089) (-194.9779, -226.922) (-195.4078, -226.7565) (-195.8386, -226.5925) (-196.2703, -226.43) (-196.703, -226.2689) (-197.1366, -226.1094) (-197.571, -225.9514) (-198.0064, -225.7948) (-198.4427, -225.6397) (-198.7925, -225.5167) (-199.0552, -225.4252) (-199.2305, -225.3645) (-199.3182, -225.3342) knots 0.10707295 0.10707295 0.10707295 0.10707295 0.10707295 0.10707295 0.11428571 0.12857143 0.14285714 0.15714286 0.17142857 0.18571429 0.2 0.21428571 0.22857143 0.24285714 0.25714286 0.27142857 0.28571429 0.3 0.31428571 0.32857143 0.34285714 0.35714286 0.37142857 0.38571429 0.4 0.41428571 0.42857143 0.44285714 0.45714286 0.47142857 0.48571429 0.5 0.51428571 0.52857143 0.54285714 0.55714286 0.57142857 0.58571429 0.6 0.61428571 0.62857143 0.64285714 0.65714286 0.67142857 0.68571429 0.7 0.71428571 0.72857143 0.74285714 0.75714286 0.77142857 0.78571429 0.8 0.81428571 0.82857143 0.84285714 0.85714286 0.87142857 0.88571429 0.9 0.91428571 0.92857143 0.94285714 0.95714286 0.97142857 0.98571429 1 1 1 1 1 1
  arc A81 (-199.3182, -225.3342) -> (-206.1003, -232.3572) centre (11.949, -436.1388) ccw
  spline S162 degree 5 poles (-206.1003, -232.3572) (-206.0669, -232.4438) (-206.0001, -232.6169) (-205.8995, -232.8763) (-205.7644, -233.2215) (-205.5942, -233.6521) (-205.4225, -234.0818) (-205.2494, -234.5105) (-205.0748, -234.9382) (-204.8988, -235.365) (-204.7213, -235.7908) (-204.5424, -236.2157) (-204.362, -236.6395) (-204.1801, -237.0623) (-203.9967, -237.484) (-203.8118, -237.9048) (-203.6254, -238.3245) (-203.4375, -238.7431) (-203.248, -239.1606) (-203.0571, -239.5771) (-202.8646, -239.9925) (-202.6706, -240.4067) (-202.475, -240.8199) (-202.2778, -241.2319) (-202.079, -241.6427) (-201.8787, -242.0524) (-201.6768, -242.4609) (-201.4733, -242.8682) (-201.2681, -243.2743) (-201.0613, -243.6791) (-200.8529, -244.0828) (-200.6428, -244.4851) (-200.431, -244.8862) (-200.2176, -245.2859) (-200.0024, -245.6844) (-199.7855, -246.0815) (-199.5669, -246.4772) (-199.3466, -246.8715) (-199.1245, -247.2645) (-198.9006, -247.656) (-198.6749, -248.046) (-198.4473, -248.4346) (-198.218, -248.8216) (-197.9868, -249.2072) (-197.7537, -249.5912) (-197.5186, -249.9735) (-197.2816, -250.3542) (-197.0427, -250.7333) (-196.8017, -251.1106) (-196.5587, -251.4862) (-196.3136, -251.86) (-196.0665, -252.232) (-195.8172, -252.6022) (-195.5659, -252.9704) (-195.3122, -253.3368) (-195.0563, -253.701) (-194.798, -254.063) (-194.5373, -254.4228) (-194.2739, -254.7803) (-194.0081, -255.1354) (-193.7397, -255.4881) (-193.4688, -255.8385) (-193.1953, -256.1865) (-192.9465, -256.4977) (-192.751, -256.738) (-192.6102, -256.9088) (-192.5253, -257.0109) (-192.4967, -257.0452) knots -1 -1 -1 -1 -1 -1 -0.98571429 -0.97142857 -0.95714286 -0.94285714 -0.92857143 -0.91428571 -0.9 -0.88571429 -0.87142857 -0.85714286 -0.84285714 -0.82857143 -0.81428571 -0.8 -0.78571429 -0.77142857 -0.75714286 -0.74285714 -0.72857143 -0.71428571 -0.7 -0.68571429 -0.67142857 -0.65714286 -0.64285714 -0.62857143 -0.61428571 -0.6 -0.58571429 -0.57142857 -0.55714286 -0.54285714 -0.52857143 -0.51428571 -0.5 -0.48571429 -0.47142857 -0.45714286 -0.44285714 -0.42857143 -0.41428571 -0.4 -0.38571429 -0.37142857 -0.35714286 -0.34285714 -0.32857143 -0.31428571 -0.3 -0.28571429 -0.27142857 -0.25714286 -0.24285714 -0.22857143 -0.21428571 -0.2 -0.18571429 -0.17142857 -0.15714286 -0.14285714 -0.12857143 -0.11428571 -0.10707295 -0.10707295 -0.10707295 -0.10707295 -0.10707295 -0.10707295
  spline S163 degree 3 poles (-192.5158, -259.1011) (-192.3804, -258.9448) (-192.2769, -258.7636) (-192.1452, -258.3717) (-192.1183, -258.1648) (-192.1426, -257.7918) (-192.1798, -257.6279) (-192.3037, -257.3178) (-192.3898, -257.1734) (-192.4967, -257.0452) knots 0 0 0 0 0.062015 0.062015 0.12403 0.12403 0.174133 0.174133 0.224236 0.224236 0.224236 0.224236
  arc A82 (-192.5158, -259.1011) -> (-197.904, -265.5226) centre (11.949, -436.1388) ccw
  spline S164 degree 3 poles (-199.9254, -265.8983) (-199.7461, -266.0011) (-199.5484, -266.0679) (-199.1385, -266.122) (-198.9302, -266.1087) (-198.5689, -266.0133) (-198.4151, -265.9454) (-198.1345, -265.7643) (-198.0094, -265.6521) (-197.904, -265.5226) knots 0 0 0 0 0.062015 0.062015 0.12403 0.12403 0.174133 0.174133 0.224236 0.224236 0.224236 0.224236
  spline S165 degree 5 poles (-199.9254, -265.8983) (-199.9641, -265.8761) (-200.0794, -265.8102) (-200.272, -265.7012) (-200.5426, -265.5504) (-200.8923, -265.3594) (-201.2825, -265.1505) (-201.6746, -264.9446) (-202.0686, -264.7415) (-202.4645, -264.5414) (-202.8622, -264.3441) (-203.2618, -264.1498) (-203.6632, -263.9583) (-204.0664, -263.7695) (-204.4712, -263.5834) (-204.8775, -263.3997) (-205.2853, -263.2186) (-205.6946, -263.0398) (-206.1053, -262.8634) (-206.5173, -262.6893) (-206.9308, -262.5175) (-207.3455, -262.3479) (-207.7616, -262.1807) (-208.179, -262.0156) (-208.5976, -261.8527) (-209.0175, -261.692) (-209.4385, -261.5333) (-209.8606, -261.3767) (-210.284, -261.2222) (-210.7084, -261.0696) (-211.1339, -260.9191) (-211.5605, -260.7706) (-211.9882, -260.624) (-212.4169, -260.4794) (-212.8467, -260.3367) (-213.2774, -260.1959) (-213.7092, -260.057) (-214.1419, -259.92) (-214.5756, -259.7848) (-215.0102, -259.6515) (-215.4457, -259.5199) (-215.8822, -259.3902) (-216.3195, -259.2623) (-216.7578, -259.1362) (-217.1969, -259.0118) (-217.6369, -258.8891) (-218.0777, -258.7683) (-218.5194, -258.6491) (-218.9618, -258.5317) (-219.4051, -258.4159) (-219.8493, -258.3019) (-220.2941, -258.1895) (-220.7398, -258.0788) (-221.1863, -257.9698) (-221.6335, -257.8625) (-222.0814, -257.7567) (-222.5302, -257.6527) (-222.9796, -257.5502) (-223.4297, -257.4494) (-223.8806, -257.3501) (-224.3322, -257.2525) (-224.7844, -257.1564) (-225.2374, -257.062) (-225.691, -256.9691) (-226.0545, -256.896) (-226.3274, -256.842) (-226.5094, -256.8062) (-226.6005, -256.7884) knots 0.10707295 0.10707295 0.10707295 0.10707295 0.10707295 0.10707295 0.11428571 0.12857143 0.14285714 0.15714286 0.17142857 0.18571429 0.2 0.21428571 0.22857143 0.24285714 0.25714286 0.27142857 0.28571429 0.3 0.31428571 0.32857143 0.34285714 0.35714286 0.37142857 0.38571429 0.4 0.41428571 0.42857143 0.44285714 0.45714286 0.47142857 0.48571429 0.5 0.51428571 0.52857143 0.54285714 0.55714286 0.57142857 0.58571429 0.6 0.61428571 0.62857143 0.64285714 0.65714286 0.67142857 0.68571429 0.7 0.71428571 0.72857143 0.74285714 0.75714286 0.77142857 0.78571429 0.8 0.81428571 0.82857143 0.84285714 0.85714286 0.87142857 0.88571429 0.9 0.91428571 0.92857143 0.94285714 0.95714286 0.97142857 0.98571429 1 1 1 1 1 1
  arc A83 (-226.6005, -256.7884) -> (-232.3391, -264.687) centre (11.949, -436.1388) ccw
  spline S166 degree 5 poles (-232.3391, -264.687) (-232.2941, -264.7681) (-232.2038, -264.9302) (-232.0681, -265.173) (-231.8863, -265.4961) (-231.6578, -265.8989) (-231.428, -266.3004) (-231.1969, -266.7009) (-230.9645, -267.1002) (-230.7308, -267.4983) (-230.4957, -267.8953) (-230.2594, -268.2911) (-230.0218, -268.6857) (-229.7828, -269.079) (-229.5425, -269.4712) (-229.3008, -269.8621) (-229.0579, -270.2517) (-228.8135, -270.6401) (-228.5678, -271.0273) (-228.3208, -271.4131) (-228.0723, -271.7976) (-227.8225, -272.1809) (-227.5713, -272.5628) (-227.3187, -272.9433) (-227.0648, -273.3225) (-226.8094, -273.7003) (-226.5525, -274.0767) (-226.2943, -274.4517) (-226.0346, -274.8253) (-225.7735, -275.1975) (-225.5109, -275.5681) (-225.2469, -275.9373) (-224.9814, -276.305) (-224.7143, -276.6712) (-224.4458, -277.0358) (-224.1758, -277.3988) (-223.9043, -277.7603) (-223.6312, -278.1201) (-223.3565, -278.4783) (-223.0803, -278.8349) (-222.8025, -279.1897) (-222.5232, -279.5428) (-222.2422, -279.8942) (-221.9595, -280.2438) (-221.6752, -280.5916) (-221.3893, -280.9375) (-221.1016, -281.2816) (-220.8122, -281.6237) (-220.5211, -281.9638) (-220.2282, -282.3019) (-219.9335, -282.6379) (-219.637, -282.9719) (-219.3386, -283.3038) (-219.0384, -283.6335) (-218.7363, -283.961) (-218.4322, -284.286) (-218.126, -284.6086) (-217.8177, -284.9286) (-217.5072, -285.2459) (-217.1945, -285.5606) (-216.8797, -285.8726) (-216.5627, -286.1818) (-216.2434, -286.4884) (-215.9536, -286.7619) (-215.7266, -286.9727) (-215.5635, -287.1222) (-215.4651, -287.2115) (-215.4321, -287.2414) knots -1 -1 -1 -1 -1 -1 -0.98571429 -0.97142857 -0.95714286 -0.94285714 -0.92857143 -0.91428571 -0.9 -0.88571429 -0.87142857 -0.85714286 -0.84285714 -0.82857143 -0.81428571 -0.8 -0.78571429 -0.77142857 -0.75714286 -0.74285714 -0.72857143 -0.71428571 -0.7 -0.68571429 -0.67142857 -0.65714286 -0.64285714 -0.62857143 -0.61428571 -0.6 -0.58571429 -0.57142857 -0.55714286 -0.54285714 -0.52857143 -0.51428571 -0.5 -0.48571429 -0.47142857 -0.45714286 -0.44285714 -0.42857143 -0.41428571 -0.4 -0.38571429 -0.37142857 -0.35714286 -0.34285714 -0.32857143 -0.31428571 -0.3 -0.28571429 -0.27142857 -0.25714286 -0.24285714 -0.22857143 -0.21428571 -0.2 -0.18571429 -0.17142857 -0.15714286 -0.14285714 -0.12857143 -0.11428571 -0.10707295 -0.10707295 -0.10707295 -0.10707295 -0.10707295 -0.10707295
  spline S167 degree 3 poles (-215.1648, -289.28) (-215.0526, -289.1064) (-214.9753, -288.9126) (-214.8994, -288.5061) (-214.9015, -288.2975) (-214.9775, -287.9316) (-215.0371, -287.7744) (-215.203, -287.4845) (-215.3083, -287.3536) (-215.4321, -287.2414) knots 0 0 0 0 0.062015 0.062015 0.12403 0.12403 0.174133 0.174133 0.224236 0.224236 0.224236 0.224236
  arc A84 (-215.1648, -289.28) -> (-219.6069, -296.3889) centre (11.949, -436.1388) ccw
  spline S168 degree 3 poles (-221.5563, -297.0423) (-221.3644, -297.1191) (-221.1594, -297.1578) (-220.7459, -297.1543) (-220.5416, -297.1122) (-220.197, -296.9674) (-220.0542, -296.8788) (-219.8015, -296.6603) (-219.6932, -296.5319) (-219.6069, -296.3889) knots 0 0 0 0 0.062015 0.062015 0.12403 0.12403 0.174133 0.174133 0.224236 0.224236 0.224236 0.224236
  spline S169 degree 5 poles (-221.5563, -297.0423) (-221.5977, -297.0257) (-221.7211, -296.9765) (-221.927, -296.8954) (-222.216, -296.7837) (-222.5888, -296.6432) (-223.0043, -296.4906) (-223.4213, -296.3413) (-223.8397, -296.195) (-224.2596, -296.0519) (-224.6809, -295.912) (-225.1036, -295.7751) (-225.5278, -295.6413) (-225.9533, -295.5105) (-226.38, -295.3825) (-226.808, -295.2573) (-227.2371, -295.1346) (-227.6672, -295.0145) (-228.0985, -294.897) (-228.5307, -294.7819) (-228.9641, -294.6693) (-229.3984, -294.5592) (-229.8337, -294.4514) (-230.27, -294.3461) (-230.7072, -294.243) (-231.1453, -294.1423) (-231.5843, -294.0437) (-232.0242, -293.9474) (-232.4649, -293.8533) (-232.9064, -293.7613) (-233.3488, -293.6715) (-233.7919, -293.5838) (-234.2358, -293.4982) (-234.6805, -293.4146) (-235.1259, -293.3331) (-235.5721, -293.2537) (-236.0189, -293.1762) (-236.4665, -293.1007) (-236.9148, -293.0272) (-237.3637, -292.9556) (-237.8133, -292.886) (-238.2636, -292.8183) (-238.7145, -292.7525) (-239.166, -292.6886) (-239.6182, -292.6265) (-240.0709, -292.5663) (-240.5243, -292.5079) (-240.9782, -292.4514) (-241.4328, -292.3967) (-241.8879, -292.3438) (-242.3435, -292.2927) (-242.7997, -292.2433) (-243.2565, -292.1957) (-243.7137, -292.1499) (-244.1715, -292.1058) (-244.6299, -292.0635) (-245.0887, -292.0229) (-245.548, -291.9839) (-246.0078, -291.9467) (-246.4681, -291.9112) (-246.9289, -291.8774) (-247.3901, -291.8452) (-247.8518, -291.8147) (-248.3139, -291.7859) (-248.684, -291.7641) (-248.9618, -291.7485) (-249.147, -291.7385) (-249.2397, -291.7335) knots 0.10707295 0.10707295 0.10707295 0.10707295 0.10707295 0.10707295 0.11428571 0.12857143 0.14285714 0.15714286 0.17142857 0.18571429 0.2 0.21428571 0.22857143 0.24285714 0.25714286 0.27142857 0.28571429 0.3 0.31428571 0.32857143 0.34285714 0.35714286 0.37142857 0.38571429 0.4 0.41428571 0.42857143 0.44285714 0.45714286 0.47142857 0.48571429 0.5 0.51428571 0.52857143 0.54285714 0.55714286 0.57142857 0.58571429 0.6 0.61428571 0.62857143 0.64285714 0.65714286 0.67142857 0.68571429 0.7 0.71428571 0.72857143 0.74285714 0.75714286 0.77142857 0.78571429 0.8 0.81428571 0.82857143 0.84285714 0.85714286 0.87142857 0.88571429 0.9 0.91428571 0.92857143 0.94285714 0.95714286 0.97142857 0.98571429 1 1 1 1 1 1
  arc A85 (-249.2397, -291.7335) -> (-253.8232, -300.3539) centre (11.949, -436.1388) ccw